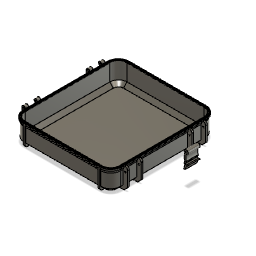
boxw-acc-vii-v15 (Autodesk Fusion 360 design; units mm, degrees)
Autodesk Fusion 360 part; units mm, degrees
sketch "Sketch1" plane through (0, 0, 0) normal (0, 1, 0) x (1, 0, 0)
  line L0 (75.5, -93) -> (-75.5, -93)
  line L1 (-85.5, -83) -> (-85.5, 83)
  line L2 (-75.5, 93) -> (75.5, 93)
  line L3 (85.5, 83) -> (85.5, -83)
  line L4 (85.5, -93) -> (-85.5, 93) construction
  line L5 (-85.5, -93) -> (85.5, 93) construction
  arc A0 (-75.5, 93) -> (-85.5, 83) centre (-75.5, 83) ccw
  arc A1 (85.5, 83) -> (75.5, 93) centre (75.5, 83) ccw
  arc A2 (75.5, -93) -> (85.5, -83) centre (75.5, -83) ccw
  arc A3 (-85.5, -83) -> (-75.5, -93) centre (-75.5, -83) ccw
  dimension "d6" = 186
  dimension "d7" = 171
  dimension "d8" = 10
  dimension "d9" = 10
  dimension "d10" = 10
  dimension "d11" = 10
  constraint horizontal L0
  constraint perpendicular L0 L1
  constraint parallel L0 L2
  constraint parallel L1 L3
  constraint coincident L4 origin
  constraint coincident L5 origin
  constraint coincident L4.end L2
  constraint coincident L4.end L1
  constraint tangent L2 A0
  constraint tangent L1 A0
  constraint coincident L5.end L2
  constraint coincident L5.end L3
  constraint tangent L2 A1
  constraint tangent L3 A1
  constraint coincident L4.start L3
  constraint coincident L4.start L0
  constraint tangent L3 A2
  constraint tangent L0 A2
  constraint coincident L5.start L0
  constraint coincident L5.start L1
  constraint tangent L0 A3
  constraint tangent L1 A3
  measures "d6" distance of L0 L2
  measures "d7" distance of L1 L3
  measures "d8" radius of A0
  measures "d9" radius of A1
  measures "d10" radius of A2
  measures "d11" radius of A3
sketch "Sketch2" plane through (0, 0, 0) normal (0, 0, 1) x (1, 0, 0)
  line L0 (0, 0) -> (85.5, 0)
  line L1 (85.5, 0) -> (85.5, 2.4)
  line L2 (92.5, 9.4) -> (92.5, 42.4)
  line L3 (92.5, 42.4) -> (93.73, 42.4)
  line L4 (93.73, 42.4) -> (93.73, 40.4)
  line L5 (93.73, 40.4) -> (95.53, 40.4)
  line L6 (95.53, 40.4) -> (95.53, 42.4)
  line L7 (95.53, 42.4) -> (96.76, 42.4)
  line L8 (96.76, 42.4) -> (96.76, 39.4)
  line L9 (95.6865, 0) -> (85.5, 0)
  line L10 (96.76, 39.4) -> (94.9, 39.4)
  line L11 (94.9, 39.4) -> (94.9, 35)
  line L12 (94.9, 35) -> (94.9, 8.4059)
  line L13 (94.9, 35) -> (96.76, 39.4)
  line L14 (92.5, 9.4) -> (85.5, 2.4)
  line L15 (86.4941, 0) -> (94.9, 8.4059)
  line L16 (95.6865, 0) -> (103.76, 8.0735)
  line L17 (96.76, 42.4) -> (98.76, 42.4)
  line L18 (103.76, 37.4) -> (103.76, 8.0735)
  arc A0 (103.76, 37.4) -> (98.76, 42.4) centre (98.76, 37.4) ccw
  circle A1 centre (99.26, 32.4) radius 1.425
  line L19 (0, 0) -> (0, 60)
  line L20 (-103.76, 37.4) -> (-103.76, 8.0735)
  line L21 (-93.73, 42.4) -> (-93.73, 40.4)
  line L22 (-94.9, 35) -> (-96.76, 39.4)
  line L23 (-92.5, 9.4) -> (-92.5, 42.4)
  line L24 (-85.5, 0) -> (-85.5, 2.4)
  line L25 (-93.73, 40.4) -> (-95.53, 40.4)
  line L26 (-86.4941, 0) -> (-94.9, 8.4059)
  line L27 (-94.9, 35) -> (-94.9, 8.4059)
  line L28 (-92.5, 9.4) -> (-85.5, 2.4)
  line L29 (-96.76, 42.4) -> (-96.76, 39.4)
  line L30 (-95.6865, 0) -> (-103.76, 8.0735)
  line L31 (-94.9, 39.4) -> (-94.9, 35)
  line L32 (-95.53, 42.4) -> (-96.76, 42.4)
  line L33 (-95.53, 40.4) -> (-95.53, 42.4)
  line L34 (-95.6865, 0) -> (-85.5, 0)
  line L35 (-96.76, 39.4) -> (-94.9, 39.4)
  line L36 (-92.5, 42.4) -> (-93.73, 42.4)
  line L37 (94.9, 39.4) -> (92.5, 39.4)
  line L38 (-94.9, 39.4) -> (-92.5, 39.4)
  circle A2 centre (-100.36, 42.4) radius 1.425
  circle A3 centre (-100.36, 42.4) radius 3.4
  line L39 (-103.76, 42.4) -> (-103.76, 37.4)
  line L40 (-96.76, 42.4) -> (-96.96, 42.4)
  line L41 (-102.7642, 39.9958) -> (-92.5, 29.7317)
  line L42 (-102.7642, 39.9958) -> (-39.091, 39.9958) construction
  line L43 (-100.36, 42.4) -> (-96.76, 42.4)
  point P0 (103.76, 42.4)
  point P1 (-103.76, 42.4)
  dimension "d12" = 85.5
  dimension "d13" = 2.4
  dimension "d15" = 1.23
  dimension "d16" = 2
  dimension "d17" = 1.8
  dimension "d18" = 2
  dimension "d20" = 3
  dimension "d23" = 4.4
  dimension "d26" = 2.4
  dimension "d27" = 7
  dimension "d28" = 7
  dimension "d29" = 42.4
  dimension "d30" = 6.5
  dimension "d61" = 7
  dimension "d62" = 5
  dimension "d63" = 2.85
  dimension "d64" = 10
  dimension "d65" = 4.5
  dimension "d129" = 1.23
  dimension "d131" = 2.4
  dimension "d137" = 2.85
  dimension "d138" = 3.6
  dimension "d139" = 6.8
  dimension "d140" = 45
  constraint coincident L0.start L19.start
  constraint horizontal L0
  constraint perpendicular L0 L1
  constraint perpendicular L2 L3
  constraint perpendicular L3 L4
  constraint perpendicular L4 L5
  constraint perpendicular L5 L6
  constraint perpendicular L6 L7
  constraint perpendicular L7 L8
  constraint perpendicular L1 L9
  constraint perpendicular L8 L10
  constraint perpendicular L10 L11
  constraint perpendicular L9 L12
  constraint coincident L9 L15.start
  constraint vertical L2
  constraint perpendicular L8 L17
  constraint perpendicular L7 L18
  constraint coincident P0 L17
  constraint coincident P0 L18
  constraint tangent L17 A0
  constraint tangent L18 A0
  constraint perpendicular L0 L19
  constraint symmetric L0.end L19 L24.start
  constraint symmetric L1.end L19 L24.end
  constraint symmetric L2.end L19 L23.end
  constraint symmetric L3.end L19 L21.start
  constraint symmetric L4.end L19 L21.end
  constraint symmetric L5.end L19 L25.end
  constraint symmetric L6.end L19 L32.start
  constraint symmetric L7.end L19 L29.start
  constraint symmetric L8.end L19 L22.end
  constraint symmetric L10.end L19 L31.start
  constraint symmetric L11.end L19 L22.start
  constraint symmetric L2.start L19 L23.start
  constraint symmetric L15.start L19 L26.start
  constraint symmetric L12.end L19 L26.end
  constraint symmetric L9.start L19 L30.start
  constraint symmetric P0 L19 P1
  constraint symmetric L16.end L19 L20.end
  constraint symmetric L18.start L19 L20.start
  constraint coincident L2 L37.end
  constraint perpendicular L2 L37
  constraint coincident L23 L38.end
  constraint perpendicular L23 L38
  constraint concentric A2 A3
  constraint coincident P1 L39.start
  constraint coincident A3 L40.end
  constraint horizontal L42
  constraint coincident A3 L41.start
  constraint tangent A3 L41
  constraint coincident L23 L41.end
  constraint coincident A2.centre A3.centre
  constraint perpendicular L29 L43
  constraint horizontal L40
  measures "d12" distance of L0.start L0.end
  measures "d13" distance of L0.end L1.end
  measures "d15" distance of L2.end L3.end
  measures "d16" distance of L3.end L4.end
  measures "d17" distance of L4.end L5.end
  measures "d18" distance of L5.end L6.end
  measures "d20" distance of L7.end L8.end
  measures "d23" distance of L10.end L11.end
  measures "d26" distance of L14 L15
  measures "d27" vertical distance of L1.end L2.start
  measures "d28" horizontal distance of L1.end L2.start
  measures "d29" distance of L0.end L7
  measures "d30" distance of L15 L16
  measures "d61" distance of L7.end P0
  measures "d62" radius of A0
  measures "d63" diameter of A1
  measures "d64" distance of L17 A1.centre
  measures "d65" distance of L18 A1.centre
  measures "d129" distance of L6 L8
  measures "d131" distance of L2 L12
  measures "d137" diameter of A2
  measures "d138" distance of L29.start A2.centre
  measures "d139" diameter of A3
  measures "d140" angle of L41 L42
extrude "Extrude1" add sketch "Sketch1" along normal blind 2.4 makes body 1
sweep "Sweep1" add profiles "Sketch2" path "Sketch1" along A2 L0 A3 L1 A0 L2 A1 L3 section 1 contours L1 L2 L9 L11 L12 L14 L15 L37 | L2 L3 L4 L5 L6 L7 L8 L10 L37 | L10 L11 L13 bodies 1
ref_plane "WorkPlane2" through (-73.5, 0, 0) normal (1, 0, 0) x (0, 1, 0)
sketch "Sketch4" plane through (-73.5, 0, 0) normal (1, 0, 0) x (0, 0, -1)
  line L0 (0, 0) -> (-93, 0)
  line L1 (-93, 0) -> (-93, 2.4)
  line L2 (-93, 2.4) -> (-100, 2.4)
  line L3 (-100, 2.4) -> (-100, 9.4)
  line L4 (-100, 9.4) -> (-93, 2.4)
  line L5 (-100, 2.4) -> (-100, 5)
  line L6 (-100, 2.4) -> (-100, 39.4)
  line L7 (-100, 39.4) -> (-104.26, 39.4)
  line L8 (-104.26, 39.4) -> (-104.26, 4.4676)
  line L9 (-99.7924, 0) -> (-93, 0)
  line L10 (-99.7924, 0) -> (-104.26, 4.4676)
  line L11 (0, 0) -> (0, 70)
  line L12 (99.7924, 0) -> (104.26, 4.4676)
  line L13 (99.7924, 0) -> (93, 0)
  line L14 (100, 2.4) -> (100, 5)
  line L15 (100, 2.4) -> (100, 39.4)
  line L16 (100, 9.4) -> (93, 2.4)
  line L17 (100, 2.4) -> (100, 9.4)
  line L18 (100, 39.4) -> (104.26, 39.4)
  line L19 (104.26, 39.4) -> (104.26, 4.4676)
  line L20 (93, 0) -> (93, 2.4)
  line L21 (93, 2.4) -> (100, 2.4)
  dimension "d47" = 93
  dimension "d48" = 2.4
  dimension "d49" = 7
  dimension "d50" = 7
  dimension "d52" = 4.26
  dimension "d53" = 6.5
  dimension "d56" = 39.4
  constraint coincident L0.start L11.start
  constraint horizontal L0
  constraint perpendicular L0 L1
  constraint perpendicular L1 L2
  constraint perpendicular L2 L3
  constraint coincident L3 L5.end
  constraint perpendicular L2 L6
  constraint perpendicular L6 L7
  constraint perpendicular L7 L8
  constraint perpendicular L1 L9
  constraint perpendicular L0 L11
  constraint symmetric L0.end L11 L13.end
  constraint symmetric L1.end L11 L16.end
  constraint symmetric L2.end L11 L14.start
  constraint symmetric L3.end L11 L16.start
  constraint symmetric L5.end L11 L14.end
  constraint symmetric L6.end L11 L15.end
  constraint symmetric L7.end L11 L18.end
  constraint symmetric L8.end L11 L12.end
  constraint symmetric L9.start L11 L12.start
  measures "d47" distance of L0.start L0.end
  measures "d48" distance of L0.end L1.end
  measures "d49" distance of L1.end L2.end
  measures "d50" distance of L2.end L3.end
  measures "d52" distance of L6.end L7.end
  measures "d53" distance of L4 L10
  measures "d56" distance of L7 L9
extrude "Extrude2" add sketch "Sketch4" along normal mid plane 3.2 bodies 1
ref_plane "WorkPlane3" through (73.5, 0, 0) normal (1, 0, 0) x (0, 1, 0)
sketch "Sketch5" plane through (73.5, 0, 0) normal (1, 0, 0) x (0, 0, -1)
  line L0 (-100, 2.4) -> (-100, 39.4)
  line L1 (-100, 9.4) -> (-93, 2.4)
  line L2 (-93, 2.4) -> (-100, 2.4)
  line L3 (-93, 0) -> (-93, 2.4)
  line L4 (-99.7924, 0) -> (-93, 0)
  line L5 (-99.7924, 0) -> (-104.26, 4.4676)
  line L6 (-104.26, 39.4) -> (-104.26, 4.4676)
  line L7 (-100, 39.4) -> (-104.26, 39.4)
  line L8 (100, 39.4) -> (104.26, 39.4)
  line L9 (104.26, 39.4) -> (104.26, 4.4676)
  line L10 (100, 2.4) -> (100, 39.4)
  line L11 (100, 9.4) -> (93, 2.4)
  line L12 (93, 2.4) -> (100, 2.4)
  line L13 (99.7924, 0) -> (104.26, 4.4676)
  line L14 (93, 0) -> (93, 2.4)
  line L15 (99.7924, 0) -> (93, 0)
extrude "Extrude3" add sketch "Sketch5" along normal mid plane 3.2 bodies 1
ref_plane "WorkPlane4" through (0, 0, -75) normal (0, 0, 1) x (1, 0, 0)
sketch "Sketch6" plane through (0, 0, -75) normal (0, 0, 1) x (1, 0, 0)
  line L0 (96.76, 42.4) -> (98.76, 42.4)
  line L1 (103.76, 37.4) -> (103.76, 8.0735)
  arc A0 (103.76, 37.4) -> (98.76, 42.4) centre (98.76, 37.4) ccw
  line L2 (95.6865, 0) -> (103.76, 8.0735)
  line L3 (95.6865, 0) -> (85.5, 0)
  line L4 (85.5, 0) -> (85.5, 2.4)
  line L5 (92.5, 9.4) -> (85.5, 2.4)
  line L6 (92.5, 9.4) -> (92.5, 42.4)
  line L7 (94.9, 39.4) -> (92.5, 39.4)
  line L8 (96.76, 39.4) -> (94.9, 39.4)
  line L9 (96.76, 42.4) -> (96.76, 39.4)
  line L10 (-92.5, 9.4) -> (-92.5, 42.4)
  line L11 (-94.9, 39.4) -> (-92.5, 39.4)
  line L12 (-96.76, 39.4) -> (-94.9, 39.4)
  line L13 (-96.76, 42.4) -> (-96.76, 39.4)
  line L14 (-103.76, 37.4) -> (-103.76, 8.0735)
  line L15 (-95.6865, 0) -> (-103.76, 8.0735)
  line L16 (-95.6865, 0) -> (-85.5, 0)
  line L17 (-85.5, 0) -> (-85.5, 2.4)
  line L18 (-92.5, 9.4) -> (-85.5, 2.4)
  circle A1 centre (99.26, 32.4) radius 1.425
  line L19 (-103.76, 42.4) -> (-103.76, 37.4)
  circle A2 centre (-100.36, 42.4) radius 3.4
  circle A3 centre (-100.36, 42.4) radius 1.425
  line L20 (-96.76, 42.4) -> (-96.96, 42.4)
  line L21 (-102.7642, 39.9958) -> (-92.5, 29.7317)
  point P0 (103.76, 42.4)
  point P1 (99.26, 32.4)
extrude "Extrude10" add sketch "Sketch6" against normal blind 3.2 bodies 1
extrude "Extrude17" add sketch "Sketch6" along normal blind 3 contours L10 L11 L12 L13 A2 L20 L21 | A2 bodies 1
ref_plane "WorkPlane5" through (0, 0, -51.4) normal (0, 0, 1) x (1, 0, 0)
sketch "Sketch7" plane through (0, 0, -51.4) normal (0, 0, 1) x (1, 0, 0)
  line L0 (-85.5, 0) -> (-85.5, 2.4)
  line L1 (-92.5, 9.4) -> (-85.5, 2.4)
  line L2 (-92.5, 9.4) -> (-92.5, 42.4)
  line L3 (-94.9, 39.4) -> (-92.5, 39.4)
  line L4 (-96.76, 39.4) -> (-94.9, 39.4)
  line L5 (-96.76, 42.4) -> (-96.76, 39.4)
  line L6 (-103.76, 37.4) -> (-103.76, 8.0735)
  line L7 (-95.6865, 0) -> (-103.76, 8.0735)
  line L8 (-95.6865, 0) -> (-85.5, 0)
  line L9 (85.5, 0) -> (85.5, 2.4)
  line L10 (92.5, 9.4) -> (85.5, 2.4)
  line L11 (92.5, 9.4) -> (92.5, 42.4)
  line L12 (94.9, 39.4) -> (92.5, 39.4)
  line L13 (96.76, 39.4) -> (94.9, 39.4)
  line L14 (96.76, 42.4) -> (96.76, 39.4)
  line L15 (96.76, 42.4) -> (98.76, 42.4)
  arc A0 (103.76, 37.4) -> (98.76, 42.4) centre (98.76, 37.4) ccw
  line L16 (103.76, 37.4) -> (103.76, 8.0735)
  line L17 (95.6865, 0) -> (103.76, 8.0735)
  line L18 (95.6865, 0) -> (85.5, 0)
  circle A1 centre (99.26, 32.4) radius 1.425
  line L19 (-103.76, 42.4) -> (-103.76, 37.4)
  circle A2 centre (-100.36, 42.4) radius 3.4
  line L20 (-96.76, 42.4) -> (-96.96, 42.4)
  circle A3 centre (-100.36, 42.4) radius 1.425
  line L21 (-102.7642, 39.9958) -> (-92.5, 29.7317)
extrude "Extrude11" add sketch "Sketch7" along normal blind 3.2 bodies 1
extrude "Extrude18" add sketch "Sketch7" against normal blind 3 contours L2 L3 L4 L5 A2 L20 L21 | A2 bodies 1
ref_plane "WorkPlane6" through (0, 0, 75) normal (0, 0, 1) x (1, 0, 0)
sketch "Sketch8" plane through (0, 0, 75) normal (0, 0, 1) x (1, 0, 0)
  line L0 (-103.76, 37.4) -> (-103.76, 8.0735)
  line L1 (-96.76, 42.4) -> (-96.76, 39.4)
  line L2 (-96.76, 39.4) -> (-94.9, 39.4)
  line L3 (-94.9, 39.4) -> (-92.5, 39.4)
  line L4 (-92.5, 9.4) -> (-92.5, 42.4)
  line L5 (-92.5, 9.4) -> (-85.5, 2.4)
  line L6 (-85.5, 0) -> (-85.5, 2.4)
  line L7 (-95.6865, 0) -> (-85.5, 0)
  line L8 (-95.6865, 0) -> (-103.76, 8.0735)
  line L9 (85.5, 0) -> (85.5, 2.4)
  line L10 (92.5, 9.4) -> (85.5, 2.4)
  line L11 (92.5, 9.4) -> (92.5, 42.4)
  line L12 (94.9, 39.4) -> (92.5, 39.4)
  line L13 (96.76, 39.4) -> (94.9, 39.4)
  line L14 (96.76, 42.4) -> (96.76, 39.4)
  line L15 (96.76, 42.4) -> (98.76, 42.4)
  arc A0 (103.76, 37.4) -> (98.76, 42.4) centre (98.76, 37.4) ccw
  line L16 (103.76, 37.4) -> (103.76, 8.0735)
  line L17 (95.6865, 0) -> (103.76, 8.0735)
  circle A1 centre (99.26, 32.4) radius 1.425
  line L18 (95.6865, 0) -> (85.5, 0)
  line L19 (-103.76, 42.4) -> (-103.76, 37.4)
  circle A2 centre (-100.36, 42.4) radius 3.4
  circle A3 centre (-100.36, 42.4) radius 1.425
  line L20 (-96.76, 42.4) -> (-96.96, 42.4)
  line L21 (-102.7642, 39.9958) -> (-92.5, 29.7317)
extrude "Extrude12" add sketch "Sketch8" along normal blind 3.2 bodies 1
extrude "Extrude19" add sketch "Sketch8" against normal blind 3 contours A2 | L1 L2 L3 L4 A2 L20 L21 bodies 1
ref_plane "WorkPlane7" through (0, 0, 51.4) normal (0, 0, 1) x (1, 0, 0)
sketch "Sketch9" plane through (0, 0, 51.4) normal (0, 0, 1) x (1, 0, 0)
  line L0 (95.6865, 0) -> (103.76, 8.0735)
  line L1 (95.6865, 0) -> (85.5, 0)
  line L2 (103.76, 37.4) -> (103.76, 8.0735)
  arc A0 (103.76, 37.4) -> (98.76, 42.4) centre (98.76, 37.4) ccw
  line L3 (96.76, 42.4) -> (98.76, 42.4)
  line L4 (96.76, 42.4) -> (96.76, 39.4)
  line L5 (96.76, 39.4) -> (94.9, 39.4)
  line L6 (94.9, 39.4) -> (92.5, 39.4)
  line L7 (92.5, 9.4) -> (92.5, 42.4)
  line L8 (92.5, 9.4) -> (85.5, 2.4)
  line L9 (85.5, 0) -> (85.5, 2.4)
  line L10 (-85.5, 0) -> (-85.5, 2.4)
  line L11 (-92.5, 9.4) -> (-85.5, 2.4)
  line L12 (-92.5, 9.4) -> (-92.5, 42.4)
  line L13 (-94.9, 39.4) -> (-92.5, 39.4)
  line L14 (-96.76, 39.4) -> (-94.9, 39.4)
  line L15 (-96.76, 42.4) -> (-96.76, 39.4)
  line L16 (-103.76, 37.4) -> (-103.76, 8.0735)
  line L17 (-95.6865, 0) -> (-103.76, 8.0735)
  line L18 (-95.6865, 0) -> (-85.5, 0)
  circle A1 centre (99.26, 32.4) radius 1.425
  line L19 (-103.76, 42.4) -> (-103.76, 37.4)
  circle A2 centre (-100.36, 42.4) radius 3.4
  circle A3 centre (-100.36, 42.4) radius 1.425
  line L20 (-96.76, 42.4) -> (-96.96, 42.4)
  line L21 (-102.7642, 39.9958) -> (-92.5, 29.7317)
  point P0 (98.76, 37.4)
extrude "Extrude13" add sketch "Sketch9" against normal blind 3.2 bodies 1
extrude "Extrude20" add sketch "Sketch9" along normal blind 3 contours L12 L13 L14 L15 A2 L20 L21 | A2 bodies 1
fillet "Fillet2" radius 1 53 edges at (75.3, 0, -93.9941) (83.274, 0, -90.774) (86.4941, 0, -80.6) (91.0903, 0, -78.2) (91.0903, 0, -75) (95.6865, 0, -76.6) (86.4941, 0, -63.2) (91.0903, 0, -51.4) (91.0903, 0, -48.2) (95.6865, 0, -49.8) (86.4941, 0, 0) (91.0903, 0, 48.2) (95.6865, 0, 49.8) (91.0903, 0, 51.4) (86.4941, 0, 63.2) (91.0903, 0, 75) (91.0903, 0, 78.2) (95.6865, 0, 76.6) (86.4941, 0, 80.6) (83.274, 0, 90.774) (75.3, 0, 93.9941) (75.1, 0, 96.8933) (73.5, 0, 99.7924) (71.9, 0, 96.8933) (0, 0, 93.9941) (-71.9, 0, 96.8933) (-73.5, 0, 99.7924) (-75.1, 0, 96.8933) (-75.3, 0, 93.9941) (-83.274, 0, 90.774) (-86.4941, 0, 80.6) (-91.0903, 0, 75) (-91.0903, 0, 78.2) (-95.6865, 0, 76.6) (-86.4941, 0, 63.2) (-91.0903, 0, 51.4) (-91.0903, 0, 48.2) (-95.6865, 0, 49.8) (-86.4941, 0, 0) (-91.0903, 0, -48.2) (-91.0903, 0, -51.4) (-95.6865, 0, -49.8) (-86.4941, 0, -63.2) (-91.0903, 0, -75) (-95.6865, 0, -76.6) (-91.0903, 0, -78.2) (-86.4941, 0, -80.6) (-83.274, 0, -90.774) (-75.3, 0, -93.9941) (0, 0, -93.9941) (-71.9, 0, -96.8933) (-75.1, 0, -96.8933) (-73.5, 0, -99.7924) on bodies 1
copy_body "Body->Comp1" bodies 1 removing the originals makes body 2 in component "BoxW"
sketch "Sketch10" plane through (0, 0, 0) normal (0, 0, 1) x (1, 0, 0)
  circle A0 centre (152.5, 40) radius 1.65
  circle A1 centre (152.5, 40) radius 4
  circle A2 centre (152.5, 60) radius 1.65
  circle A3 centre (152.5, 60) radius 4
  arc A4 (152.5, 60) -> (152.5, 40) centre (172.1161, 50) ccw
  arc A5 (151.0745, 60.7267) -> (151.0745, 39.2733) centre (172.1161, 50) ccw
  arc A6 (153.9344, 59.2688) -> (153.9344, 40.7312) centre (172.1161, 50) ccw
  line L0 (153.5161, 38.7) -> (156.2829, 38.7)
  line L1 (152.5, 40) -> (149.0845, 29.9809)
  circle A7 centre (149.0845, 29.9809) radius 1.6
  line L2 (150.9856, 40.5163) -> (147.5701, 30.4972)
  line L3 (154.0144, 39.4837) -> (150.5989, 29.4647)
  line L4 (152.4984, 41.65) -> (152.6105, 43.9985)
  dimension "d98" = 3.3
  dimension "d99" = 8
  dimension "d100" = 20
  dimension "d101" = 3.3
  dimension "d102" = 8
  dimension "d103" = 1.6
  dimension "d104" = -1.61
  dimension "d105" = 3.2
  dimension "d106" = 1.6
  dimension "d107" = -1.6
  constraint concentric A0 A1
  constraint coincident A0.centre A1.centre
  constraint coincident A2.centre A3.centre
  constraint concentric A2 A3
  constraint coincident A0 L0.start
  constraint coincident A1 L0.end
  constraint coincident L1.end A7.centre
  constraint coincident A0 L4.start
  constraint coincident A6 L4.end
  constraint coincident A1 L4.end
  measures "d98" diameter of A0
  measures "d99" diameter of A1
  measures "d100" distance of A0.centre A2.centre
  measures "d101" diameter of A2
  measures "d102" diameter of A3
  measures "d105" diameter of A7
extrude "Extrude15" add sketch "Sketch10" along normal mid plane 23.2 separate body contours A0 A1 A4 L4 | A1 A3 A4 A6 | A0 A1 L0 L1 L3 | A1 L0 L3 | A0 A1 A4 A5 L2 | A1 A3 A4 A5 | A2 A3 A5 A6 | A2 A3 A4 A6 | A0 A1 A5 L1 L2 | A1 L1 A7 L3 | A1 A5 L2 | A2 A3 A4 A5 | A1 L1 A7 L2 | A7 makes body 3
copy_body "Body->Comp3" bodies 3 removing the originals makes body 4 in component "Box Latch"
component "BoxW" placed x (1, 0, 0) y (0, 1, 0) z (0, 0, 1) at (0, 0, 0)
component "Box Latch" placed x (1, 0, 0) y (0, 1, 0) z (0, 0, 1) at (0, 0, 0)
equation "width = 185 mm" comment "Min=60 (Outer dimension + 22.4mm)"
equation "lengh = 200 mm" comment "Min=120 (Outer dimension + 8.4mm)"
equation "hight = 40 mm" comment "Min=20"
equation "d6 = lengh - 14 mm"
equation "d7 = width - 14 mm"
equation "d8 = rcorner"
equation "d9 = rcorner"
equation "d10 = rcorner"
equation "d11 = rcorner"
equation "d12 = width * 0.5 - 7 mm"
equation "d13 = tbox"
equation "d26 = tbox"
equation "d29 = hight + tbox"
equation "d31 = tbox"
equation "d46 = 19 mm - width * 0.5"
equation "d47 = lengh * 0.5 - 7 mm"
equation "d48 = tbox"
equation "d54 = trib / 2"
equation "d56 = hight - 3 mm + tbox"
equation "d57 = width * 0.5 - 19 mm"
equation "d58 = trib / 2"
equation "d60 = phinge - lengh * 0.5"
equation "d63 = screwhole"
equation "d68 = 30 mm - 2 * trib"
equation "d71 = lengh * 0.5 - phinge"
equation "d72 = 2 * trib - 30 mm"
equation "d81 = -trib"
equation "d83 = trib"
equation "d85 = trib"
equation "d87 = -trib"
equation "d108 = ( 30 mm - 2 * trib ) / 2 - 0.2 mm"
equation "screwhole = 2.85 mm" comment "For M3 screws"
equation "rcorner = 10 mm" comment "Min=1 Max=10"
equation "phinge = 25 mm" comment "Position of hinge and latch from lengh dimension"
equation "d131 = tbox"
equation "tbox = 2.4 mm" comment "Min=2 Max=4.2 Box thickness"
equation "trib = 3.2 mm" comment "Min=2.4 Max=3.6 Rib thickness"
equation "d137 = screwhole"
named bodies: "Box Waterproof", "BoxW", "Latch", "Box Latch"
